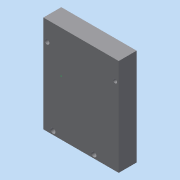
# Autodesk Inventor part: arduino
Saved by Autodesk Inventor 2015 (Build 190159000, 159)
## iProperties
Created: 2015-06-23
Part Number: arduino
Material: Generic
Document SubType Name: Modeling
Designer: Rahul
Density: 1 g/cm^3
Appearance: Default
Author: Rahul
Autodesk Inventor part; units mm, degrees
ref_plane "YZ Plane" through (0, 0, 0) normal (1, 0, 0) x (0, 1, 0)
ref_plane "XZ Plane" through (0, 0, 0) normal (0, 1, 0) x (-1, 0, 0)
ref_plane "XY Plane" through (0, 0, 0) normal (0, 0, 1) x (1, 0, 0)
sketch "Sketch1" plane through (0, 0, 0) normal (0, 0, 1) x (1, 0, 0)
  line L0 (-12.6883, 29.4299) -> (40.4231, 29.4299)
  line L1 (40.4231, 29.4299) -> (40.4231, -38.8199)
  line L2 (40.4231, -38.8199) -> (-12.6883, -38.8199)
  line L3 (-12.6883, -38.8199) -> (-12.6883, 29.4299)
  point P0 (0, 0)
  dimension "d0" = 68.2498
  dimension "d1" = 53.1114
  constraints: 8 end point, 2 parallel, 1 horizontal, 1 perpendicular
  measures "d0" distance of L0.end L1.end
  measures "d1" distance of L0.start L0.end
extrude "Extrusion1" add sketch "Sketch1" along normal blind 12.6492
sketch "Sketch2" plane through (0, 0, 12.6492) normal (0, 0, 1) x (1, 0, 0)
  line L0 (40.4231, -38.8199) -> (40.4231, 29.4299) projected
  circle A0 centre (-5.9065, -36.2799) radius 1.7526
  line L1 (-12.6883, -38.8199) -> (-12.6883, 29.4299) projected
  circle A1 centre (-10.1483, 15.9171) radius 1.7018
  line L2 (40.4231, 29.4299) -> (-12.6883, 29.4299) projected
  circle A2 centre (37.8831, 15.9171) radius 1.3716
  line L3 (-12.6883, -38.8199) -> (40.4231, -38.8199) projected
  point P0 (0, 0)
  dimension "d6" = 6.7818
  dimension "d7" = 3.5052
  dimension "d8" = 13.5128
  dimension "d9" = 3.4036
  dimension "d10" = 2.7432
  dimension "d18" = 2.54
  dimension "d21" = 2.54
  dimension "d22" = 2.54
  constraints: 3 centre point
  measures "d6" distance from line of L1 A0.centre
  measures "d7" diameter of A0
  measures "d8" distance from line of A1.centre L2
  measures "d9" diameter of A1
  measures "d10" diameter of A2
  measures "d18" distance from line of L1 A1.centre
  measures "d21" distance from line of L3 A0.centre
  measures "d22" distance from line of L0 A2.centre
extrude "Extrusion2" cut sketch "Sketch2" against normal blind 12.7 contours A1
sketch "Sketch3" plane through (0, 0, 12.6492) normal (0, 0, 1) x (1, 0, 0)
  circle A0 centre (22.9225, -36.2799) radius 1.7399
  line L0 (40.4231, -38.8199) -> (40.4231, 29.4299) projected
  line L1 (-12.6883, -38.8199) -> (40.4231, -38.8199) projected
  point P0 (0, 0)
  dimension "d13" = 17.5006
  dimension "d14" = 3.4798
  dimension "d15" = 2.54
  constraints: 1 centre point
  measures "d13" distance from line of L0 A0.centre
  measures "d14" diameter of A0
  measures "d15" distance from line of L1 A0.centre
extrude "Extrusion3" cut sketch "Sketch3" against normal blind 12.7
sketch "Sketch4" plane through (0, 0, 12.6492) normal (0, 0, 1) x (1, 0, 0)
  point P0 (0, 0)
extrude "Extrusion4" cut sketch "Sketch2" against normal blind 12.7 contours A0
extrude "Extrusion5" cut sketch "Sketch2" against normal blind 12.7 contours A2
body "Solid1"
